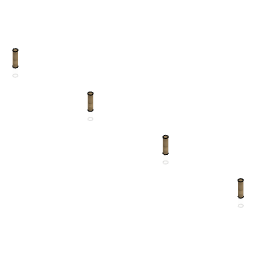
Dowels Set (Autodesk Fusion 360 design; units mm, degrees)
description: Dowel
part number: D8x30
Autodesk Fusion 360 part; units mm, degrees
sketch "Sketch1" plane through (0, 0, 0) normal (0, 0, 1) x (1, 0, 0)
  line L0 (310, 9) -> (-310, 9)
  line L1 (-310, 9) -> (-310, -9)
  line L2 (-310, -9) -> (310, -9)
  line L3 (310, -9) -> (310, 9)
  line L4 (310, 9) -> (-310, -9) construction
  line L5 (-310, 9) -> (310, -9) construction
  line L6 (-310, 0) -> (310, 0) construction
  circle A0 centre (-240, 0) radius 4
  dimension "d9" = 620
  dimension "d10" = 18
  dimension "d11" = 8
  dimension "d12" = 70
  constraint horizontal L0
  constraint perpendicular L0 L1
  constraint parallel L0 L2
  constraint parallel L1 L3
  constraint coincident L4 origin
  constraint coincident L5 origin
  constraint midpoint L1 L6.start
  constraint midpoint L3 L6.end
  constraint coincident L6 A0.centre
  measures "d9" distance of L1.end L2.end
  measures "d10" distance of L0.end L1.end
  measures "d11" diameter of A0
  measures "d12" distance of L6.start A0.centre
extrude "Extrude1" add sketch "Sketch1" along normal blind 13 and the other way blind 17 contours A0 makes body 1
extrude "Extrude2" add sketch "Sketch1" along normal blind 13 and the other way blind 34 separate body contours A0 makes body 2
copy_body "Body->Comp1" bodies 1 removing the originals makes body 3 in component "Dowel"
copy_body "CutPasteBodies1" bodies 2 removing the originals makes body 4 in component "Dowel"
pattern_linear "00000000-0000-0000-0000-000000000000" [suppressed]
component "Dowel" placed x (1, 0, 0) y (0, 1, 0) z (0, 0, 1) at (0, 0, 0)
component "Dowel" placed x (1, 0, 0) y (0, 1, 0) z (0, 0, 1) at (160, 0, 0)
component "Dowel" placed x (1, 0, 0) y (0, 1, 0) z (0, 0, 1) at (320, 0, 0)
component "Dowel" placed x (1, 0, 0) y (0, 1, 0) z (0, 0, 1) at (480, 0, 0)
equation "ContactPatchLength = 620 mm" comment "Driven length"
equation "ContactPatchWidth = 18 mm" comment "Pillar Board Thickness"
equation "MinFromEdge = 20 mm"
equation "StepBetweenDowels = 160 mm"
equation "DowelDistributionLength = ContactPatchLength - MinFromEdge * 2"
equation "DowelNo = floor(DowelDistributionLength / StepBetweenDowels) + 1"
equation "DistributionLength = StepBetweenDowels * ( DowelNo - 1 )"
equation "FromEdge = ( ContactPatchLength - DistributionLength ) / 2"
equation "d9 = ContactPatchLength"
equation "d10 = ContactPatchWidth"
equation "d11 = DowelDia"
equation "d12 = FromEdge"
equation "d15 = 30 mm - 13 mm"
equation "d25 = DowelNo"
equation "d27 = StepBetweenDowels"
equation "DowelDia = 8 mm"
named bodies: "Dowel", "Hole"
